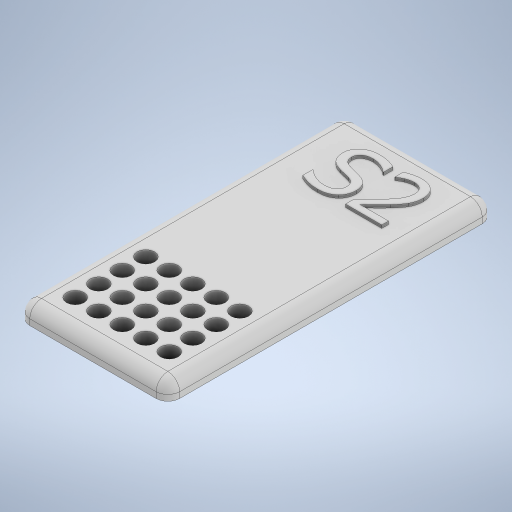
# Autodesk Inventor part: sensor2
Saved by Autodesk Inventor 2024 (Build 280153000, 153)
## iProperties
Created: 2024-03-11
Part Number: sensor2
Material: Generic
Document SubType Name: Modeling
Designer: quinten
Density: 1 g/cm^3
Appearance: Default
Author: quinten
Autodesk Inventor part; units mm, degrees
ref_plane "YZ Plane" through (0, 0, 0) normal (1, 0, 0) x (0, 1, 0)
ref_plane "XZ Plane" through (0, 0, 0) normal (0, 1, 0) x (-1, 0, 0)
ref_plane "XY Plane" through (0, 0, 0) normal (0, 0, 1) x (1, 0, 0)
sketch "Sketch1" plane through (0, 0, 0) normal (0, 1, 0) x (-1, 0, 0)
  line L0 (0, 0) -> (21.5, 0)
  line L1 (21.5, 0) -> (21.5, -51.5)
  line L2 (21.5, -51.5) -> (0, -51.5)
  line L3 (0, -51.5) -> (0, 0)
  line L4 (23.5, 2) -> (-2, 2)
  line L5 (-2, 2) -> (-2, -53.5)
  line L6 (-2, -53.5) -> (23.5, -53.5)
  line L7 (23.5, -53.5) -> (23.5, 2)
  line L8 (10.75, 0) -> (10.75, -51.5) construction
  circle A0 centre (10.75, -3) radius 1.5
  line L9 (0, -3) -> (21.5, -3) construction
  circle A1 centre (14.75, -3) radius 1.5
  circle A2 centre (18.75, -3) radius 1.5
  circle A3 centre (6.75, -3) radius 1.5
  circle A4 centre (2.75, -3) radius 1.5
  circle A5 centre (18.75, -7) radius 1.5
  circle A6 centre (14.75, -7) radius 1.5
  circle A7 centre (10.75, -7) radius 1.5
  circle A8 centre (6.75, -7) radius 1.5
  circle A9 centre (2.75, -7) radius 1.5
  circle A10 centre (18.75, -11) radius 1.5
  circle A11 centre (14.75, -11) radius 1.5
  circle A12 centre (10.75, -11) radius 1.5
  circle A13 centre (6.75, -11) radius 1.5
  circle A14 centre (2.75, -11) radius 1.5
  circle A15 centre (18.75, -15) radius 1.5
  circle A16 centre (14.75, -15) radius 1.5
  circle A17 centre (10.75, -15) radius 1.5
  circle A18 centre (6.75, -15) radius 1.5
  circle A19 centre (2.75, -15) radius 1.5
  point P0 (10.75, -3)
  point P1 (10.75, -7)
  point P2 (10.75, -11)
  point P3 (10.75, -15)
  dimension "d0" = 21.5
  dimension "d1" = 51.5
  dimension "d2" = 2
  dimension "d3" = 2
  dimension "d4" = 2
  dimension "d5" = 2
  dimension "d6" = 3
  dimension "d8" = 3
  dimension "d9" = 3
  dimension "d10" = 3
  dimension "d11" = 3
  dimension "d12" = 3
  dimension "d13" = 4
  dimension "d14" = 4
  dimension "d15" = 4
  dimension "d16" = 4
  dimension "d19" = 4
  constraints: 20 centre point, 20 end point, 7 point on line, 4 midpoint, 4 parallel, 3 perpendicular, 2 horizontal, 1 vertical, 33 other
  measures "d0" distance of L1.end L2.end
  measures "d1" distance of L0.end L1.end
  measures "d2" distance between parallel lines of L7 L1
  measures "d3" distance between parallel lines of L0 L4
  measures "d4" distance between parallel lines of L3 L5
  measures "d5" distance between parallel lines of L6 L2
  measures "d6" diameter of A0
  measures "d8" distance between parallel lines of L0 L9
  measures "d9" diameter of A1
  measures "d10" diameter of A2
  measures "d11" diameter of A3
  measures "d12" diameter of A4
  measures "d13" distance of point (10.75, -3) A3.centre
  measures "d14" distance of A3.centre A4.centre
  measures "d15" distance of A1.centre point (10.75, -3)
  measures "d16" distance of A2.centre A1.centre
  measures "d19" distance of A2.centre A5.centre
extrude "Extrusion1" add sketch "Sketch1" along normal blind 3 contours L0 L1 L2 L3 | L7 L6 L5 L4
fillet "Fillet1" radius 2 8 edges at (-23.5, 3, -25.75) (-10.75, 3, 2) (-23.5, 1.5, 2) (2, 1.5, 2) (2, 3, -25.75) (-10.75, 3, -53.5) (-23.5, 1.5, -53.5) (2, 1.5, -53.5)
sketch "Sketch2" plane through (0, 3, 0) normal (0, 1, 0) x (1, 0, 0)
  line L0 (-17.4247, 49.4836) -> (-8.1758, 49.4836) construction
  line L1 (-8.1758, 49.4836) -> (-8.1758, 43.1661) construction
  line L2 (-8.1758, 43.1661) -> (-17.4247, 43.1661) construction
  line L3 (-17.4247, 43.1661) -> (-17.4247, 49.4836) construction
  spline S0 degree 2 poles (-13.624, 39.0946) (-14.7099, 39.0946) (-16.2334, 39.5484) (-16.906, 39.8726) knots 0 0 0 1 2 2 2
  line L4 (-16.906, 39.8726) -> (-16.906, 41.5419)
  line L5 (-16.906, 41.5419) -> (-16.8088, 41.5419)
  spline S1 degree 2 poles (-16.8088, 41.5419) (-16.1524, 40.9261) (-14.4911, 40.2453) (-13.7213, 40.2453) knots 0 0 0 1 2 2 2
  spline S2 degree 2 poles (-13.7213, 40.2453) (-12.6192, 40.2453) (-11.4928, 41.1611) (-11.4928, 41.9147) knots 0 0 0 1 2 2 2
  spline S3 degree 2 poles (-11.4928, 41.9147) (-11.4928, 42.5144) (-12.0843, 43.2599) (-12.7245, 43.4463) knots 0 0 0 1 2 2 2
  spline S4 degree 2 poles (-12.7245, 43.4463) (-13.1864, 43.576) (-13.9563, 43.7543) (-14.5317, 43.9001) knots 0 0 0 1 2 2 2
  spline S5 degree 2 poles (-14.5317, 43.9001) (-15.0503, 44.0379) (-15.8688, 44.4512) (-16.1848, 44.7834) knots 0 0 0 1 2 2 2
  spline S6 degree 2 poles (-16.1848, 44.7834) (-16.4928, 45.1157) (-16.8331, 46.0071) (-16.8331, 46.5906) knots 0 0 0 1 2 2 2
  spline S7 degree 2 poles (-16.8331, 46.5906) (-16.8331, 47.8061) (-14.9368, 49.4512) (-13.4701, 49.4512) knots 0 0 0 1 2 2 2
  spline S8 degree 2 poles (-13.4701, 49.4512) (-12.6273, 49.4512) (-11.1362, 49.1189) (-10.496, 48.8029) knots 0 0 0 1 2 2 2
  line L6 (-10.496, 48.8029) -> (-10.496, 47.2146)
  line L7 (-10.496, 47.2146) -> (-10.5932, 47.2146)
  spline S9 degree 2 poles (-10.5932, 47.2146) (-11.0714, 47.6522) (-12.5624, 48.3005) (-13.3809, 48.3005) knots 0 0 0 1 2 2 2
  spline S10 degree 2 poles (-13.3809, 48.3005) (-14.3047, 48.3005) (-15.4474, 47.4334) (-15.4474, 46.7283) knots 0 0 0 1 2 2 2
  spline S11 degree 2 poles (-15.4474, 46.7283) (-15.4474, 46.0962) (-14.7748, 45.3426) (-14.1427, 45.1724) knots 0 0 0 1 2 2 2
  spline S12 degree 2 poles (-14.1427, 45.1724) (-13.7213, 45.059) (-12.4976, 44.7672) (-12.0924, 44.6457) knots 0 0 0 1 2 2 2
  spline S13 degree 2 poles (-12.0924, 44.6457) (-11.0633, 44.3296) (-10.107, 43.0573) (-10.107, 42.1254) knots 0 0 0 1 2 2 2
  spline S14 degree 2 poles (-10.107, 42.1254) (-10.107, 41.5338) (-10.5851, 40.3993) (-11.0146, 40.0022) knots 0 0 0 1 2 2 2
  spline S15 degree 2 poles (-11.0146, 40.0022) (-11.4928, 39.5646) (-12.7083, 39.0946) (-13.624, 39.0946) knots 0 0 0 1 2 2 2
  line L8 (-2.8704, 39.2729) -> (-9.0373, 39.2729)
  line L9 (-9.0373, 39.2729) -> (-9.0373, 40.691)
  spline S16 degree 2 poles (-9.0373, 40.691) (-8.3728, 41.315) (-7.1897, 42.4739) (-6.6224, 43.0979) knots 0 0 0 1 2 2 2
  spline S17 degree 2 poles (-6.6224, 43.0979) (-5.4798, 44.3539) (-4.6451, 45.8612) (-4.6451, 46.6635) knots 0 0 0 1 2 2 2
  spline S18 degree 2 poles (-4.6451, 46.6635) (-4.6451, 47.0849) (-4.9044, 47.717) (-5.1394, 47.9196) knots 0 0 0 1 2 2 2
  spline S19 degree 2 poles (-5.1394, 47.9196) (-5.3744, 48.1222) (-5.9903, 48.3248) (-6.3631, 48.3248) knots 0 0 0 1 2 2 2
  spline S20 degree 2 poles (-6.3631, 48.3248) (-6.7197, 48.3248) (-7.449, 48.1465) (-7.7812, 48.0087) knots 0 0 0 1 2 2 2
  spline S21 degree 2 poles (-7.7812, 48.0087) (-8.0649, 47.8953) (-8.5916, 47.5711) (-8.7537, 47.4577) knots 0 0 0 1 2 2 2
  line L10 (-8.7537, 47.4577) -> (-8.8266, 47.4577)
  line L11 (-8.8266, 47.4577) -> (-8.8266, 48.8839)
  spline S22 degree 2 poles (-8.8266, 48.8839) (-8.4133, 49.0865) (-6.9304, 49.4836) (-6.2659, 49.4836) knots 0 0 0 1 2 2 2
  spline S23 degree 2 poles (-6.2659, 49.4836) (-4.8639, 49.4836) (-3.2837, 48.0006) (-3.2837, 46.7364) knots 0 0 0 1 2 2 2
  spline S24 degree 2 poles (-3.2837, 46.7364) (-3.2837, 46.1449) (-3.5592, 45.1562) (-3.8023, 44.7348) knots 0 0 0 1 2 2 2
  spline S25 degree 2 poles (-3.8023, 44.7348) (-4.0454, 44.2972) (-4.7505, 43.4382) (-5.1394, 43.0249) knots 0 0 0 1 2 2 2
  spline S26 degree 2 poles (-5.1394, 43.0249) (-5.7715, 42.3361) (-7.3193, 40.8612) (-7.7812, 40.4317) knots 0 0 0 1 2 2 2
  line L12 (-7.7812, 40.4317) -> (-2.8704, 40.4317)
  line L13 (-2.8704, 40.4317) -> (-2.8704, 39.2729)
  point P0 (0, 0)
  constraints: 2 other
extrude "Extrusion2" add sketch "Sketch2" along normal blind 0.5
equation "\"d8\" = d6"
equation "\"d9\" = d11"
equation "\"d10\" = d11"
equation "\"d11\" = d6"
equation "\"d12\" = d11"
equation "\"d14\" = d13"
equation "\"d15\" = d13"
equation "\"d16\" = d15"
body "Solid1"
